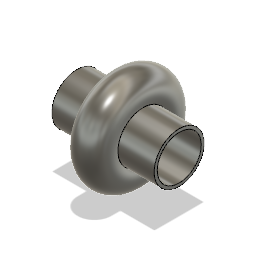
Table_13p3_Problem_6a (Autodesk Fusion 360 design; units mm, degrees)
Autodesk Fusion 360 part; units mm, degrees
sketch "Sketch1" plane through (0, 0, 0) normal (0, 0, 1) x (1, 0, 0)
  line L0 (0, 0) -> (65.3209, 0) construction
  line L1 (0, 0) -> (0, 62.8558) construction
  arc A0 (15.3209, 30) -> (0, 62.8558) centre (0, 42.8558) ccw construction
  line L2 (15.3209, 30) -> (65.3209, 30) construction
  line L3 (65.3209, 30) -> (65.3209, 0) construction
  arc A1 (10.164, 28) -> (0, 60.8558) centre (0, 42.8558) ccw
  line L4 (10.164, 28) -> (65.3209, 28)
  line L5 (19.1351, 32) -> (65.3209, 32)
  arc A2 (19.1351, 32) -> (0, 64.8558) centre (0, 42.8558) ccw
  line L6 (65.3209, 32) -> (65.3209, 28)
  line L7 (0, 42.8558) -> (15.3209, 30) construction
  line L8 (-65.3209, 32) -> (-65.3209, 28)
  line L9 (-19.1351, 32) -> (-65.3209, 32)
  line L10 (-10.164, 28) -> (-65.3209, 28)
  arc A3 (0, 60.8558) -> (-10.164, 28) centre (0, 42.8558) ccw
  arc A4 (0, 64.8558) -> (-19.1351, 32) centre (0, 42.8558) ccw
  dimension "Toroid_Radius" = 20
  dimension "Extension_Length" = 50
  dimension "Pipe_Radius" = 30
  dimension "Pipe_Thickness_1" = 2
  dimension "Pipe_Thickness_2" = 2
  dimension "Toroid_Half_Angle" = 130
  constraint coincident L0.start L1.start
  constraint horizontal L0
  constraint perpendicular L0 L1
  constraint coincident L1 A0.centre
  constraint coincident L1.end A0.end
  constraint perpendicular L1 L2
  constraint vertical L3
  constraint perpendicular L4 L6
  constraint coincident A0.centre A1.centre
  constraint symmetric L1 A1.end A3.start
  constraint symmetric L1 A1.start L10.start
  constraint symmetric L1 A1 A3
  constraint symmetric L1 L4.end L8.end
  constraint symmetric L1 L5.start L9.start
  constraint symmetric L1 L5.end L8.start
  constraint symmetric L1 A2.end A4.start
  constraint symmetric L1 A2 A4
  measures "Toroid_Radius" radius of A0
  measures "Extension_Length" distance of A0.start L2.end
  measures "Pipe_Radius" distance of L0.end L2.end
  measures "Toroid_Half_Angle" angle of L1 L7
revolve "Revolve1" add sketch "Sketch1" angle 360 about axis through (0, 0, 0) along (1, 0, 0)
